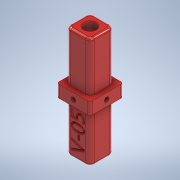
# Autodesk Inventor part: Supports
Saved by Autodesk Inventor 2020 (Build 240168000, 168)
## iProperties
Created: 2019-07-12
Part Number: Supports
Material: PBT Plastic
Document SubType Name: Modeling
Designer: steele
Density: 1.31 g/cm^3
Appearance: Orange-Red
Author: steele
Autodesk Inventor part; units mm, degrees
ref_plane "YZ Plane" through (0, 0, 0) normal (1, 0, 0) x (0, 1, 0)
ref_plane "XZ Plane" through (0, 0, 0) normal (0, 1, 0) x (-1, 0, 0)
ref_plane "XY Plane" through (0, 0, 0) normal (0, 0, 1) x (1, 0, 0)
sketch "Sketch1" plane through (0, 0, 0) normal (0, 1, 0) x (-1, 0, 0)
  line L0 (11.43, 11.43) -> (-11.43, 11.43)
  line L1 (-11.43, 11.43) -> (-11.43, -11.43)
  line L2 (-11.43, -11.43) -> (11.43, -11.43)
  line L3 (11.43, -11.43) -> (11.43, 11.43)
  line L4 (11.43, 11.43) -> (-11.43, -11.43) construction
  line L5 (-11.43, 11.43) -> (11.43, -11.43) construction
  point P0 (0, 0)
  dimension "outerWidth" = 22.86
  dimension "outerLength" = 22.86
  constraints: 12 end point, 2 midpoint, 2 parallel, 1 horizontal, 1 perpendicular
  measures "outerWidth" distance of L0.start L0.end
  measures "outerLength" distance of L1.end L0.end
extrude "CenterPortion" add sketch "Sketch1" along normal mid plane 8.382
sketch "Sketch2" plane through (0, 0, 0) normal (0, 1, 0) x (-1, 0, 0)
  line L0 (8.255, 8.255) -> (-8.255, 8.255)
  line L1 (-8.255, 8.255) -> (-8.255, -8.255)
  line L2 (-8.255, -8.255) -> (8.255, -8.255)
  line L3 (8.255, -8.255) -> (8.255, 8.255)
  line L4 (8.255, 8.255) -> (-8.255, -8.255) construction
  line L5 (-8.255, 8.255) -> (8.255, -8.255) construction
  point P0 (0, 0)
  dimension "innerWidth" = 16.51
  dimension "innerLength" = 16.51
  constraints: 12 end point, 2 midpoint, 2 parallel, 1 horizontal, 1 perpendicular
  measures "innerWidth" distance of L0.start L0.end
  measures "innerLength" distance of L1.end L0.end
extrude "OuterPortion" add sketch "Sketch2" along normal mid plane 76.2
sketch "Sketch3" plane through (-8.255, -4.191, 8.255) normal (0, 0, 1) x (1, 0, 0)
  line L0 (0, -33.909) -> (16.51, -33.909) construction
  line L1 (12.7, -33.909) -> (12.7, 0) construction
  line L2 (19.685, 0) -> (-3.175, 0) construction
  line L3 (16.51, -33.909) -> (16.51, 0) projected
  line L4 (3.81, -22.1451) -> (12.7, -25.2069)
  line L5 (12.7, -25.2069) -> (12.7, -26.4821)
  line L6 (12.7, -26.4821) -> (3.81, -29.5439)
  line L7 (3.81, -29.5439) -> (3.81, -28.2759)
  line L8 (3.81, -28.2759) -> (11.1943, -25.8121)
  line L9 (11.1943, -25.8121) -> (3.81, -23.3482)
  line L10 (3.81, -23.3482) -> (3.81, -22.1451)
  line L11 (9.35, -18.19) -> (9.35, -21.5544)
  line L12 (9.35, -21.5544) -> (8.2694, -21.5544)
  line L13 (8.2694, -21.5544) -> (8.2694, -18.19)
  line L14 (8.2694, -18.19) -> (9.35, -18.19)
  spline S0 degree 2 poles (8.255, -11.4757) (10.6468, -11.4757) (12.8873, -12.8661) (12.8873, -14.3142) knots 0 0 0 1 2 2 2
  spline S1 degree 2 poles (12.8873, -14.3142) (12.8873, -15.7838) (10.6036, -17.1598) (8.2622, -17.1598) knots 0 0 0 1 2 2 2
  spline S2 degree 2 poles (8.2622, -17.1598) (5.856, -17.1598) (3.6299, -15.7694) (3.6299, -14.3142) knots 0 0 0 1 2 2 2
  spline S3 degree 2 poles (3.6299, -14.3142) (3.6299, -12.8517) (5.9352, -11.4757) (8.255, -11.4757) knots 0 0 0 1 2 2 2
  spline S4 degree 2 poles (10.9638, -13.003) (10.5243, -12.8301) (9.1699, -12.686) (8.255, -12.686) knots 0 0 0 1 2 2 2
  spline S5 degree 2 poles (8.255, -12.686) (7.3401, -12.686) (5.9929, -12.8301) (5.539, -13.0102) knots 0 0 0 1 2 2 2
  spline S6 degree 2 poles (5.539, -13.0102) (5.0851, -13.1903) (4.6169, -13.8171) (4.6169, -14.3142) knots 0 0 0 1 2 2 2
  spline S7 degree 2 poles (4.6169, -14.3142) (4.6169, -14.8112) (5.0851, -15.4524) (5.5534, -15.6397) knots 0 0 0 1 2 2 2
  spline S8 degree 2 poles (5.5534, -15.6397) (6.0073, -15.8198) (7.3905, -15.9495) (8.2622, -15.9495) knots 0 0 0 1 2 2 2
  spline S9 degree 2 poles (8.2622, -15.9495) (9.1988, -15.9495) (10.4523, -15.8342) (10.9422, -15.6469) knots 0 0 0 1 2 2 2
  spline S10 degree 2 poles (10.9422, -15.6469) (11.4032, -15.474) (11.9003, -14.8329) (11.9003, -14.3142) knots 0 0 0 1 2 2 2
  spline S11 degree 2 poles (11.9003, -14.3142) (11.9003, -13.8243) (11.4321, -13.1831) (10.9638, -13.003) knots 0 0 0 1 2 2 2
  spline S12 degree 2 poles (9.8759, -4.9487) (10.5171, -4.9487) (11.6122, -5.3593) (12.0156, -5.7339) knots 0 0 0 1 2 2 2
  spline S13 degree 2 poles (12.0156, -5.7339) (12.419, -6.1086) (12.8873, -7.2252) (12.8873, -7.9168) knots 0 0 0 1 2 2 2
  spline S14 degree 2 poles (12.8873, -7.9168) (12.8873, -8.5508) (12.6063, -9.7899) (12.383, -10.2438) knots 0 0 0 1 2 2 2
  line L15 (12.383, -10.2438) -> (11.1223, -10.2438)
  line L16 (11.1223, -10.2438) -> (11.1223, -10.1573)
  spline S15 degree 2 poles (11.1223, -10.1573) (11.2231, -10.0204) (11.4825, -9.5089) (11.5978, -9.1992) knots 0 0 0 1 2 2 2
  spline S16 degree 2 poles (11.5978, -9.1992) (11.7202, -8.8462) (11.8571, -8.2626) (11.8571, -7.8952) knots 0 0 0 1 2 2 2
  spline S17 degree 2 poles (11.8571, -7.8952) (11.8571, -7.535) (11.5978, -6.8578) (11.3168, -6.6129) knots 0 0 0 1 2 2 2
  spline S18 degree 2 poles (11.3168, -6.6129) (11.0502, -6.3895) (10.3442, -6.159) (9.8687, -6.159) knots 0 0 0 1 2 2 2
  spline S19 degree 2 poles (9.8687, -6.159) (9.3933, -6.159) (8.7881, -6.4183) (8.5864, -6.6633) knots 0 0 0 1 2 2 2
  spline S20 degree 2 poles (8.5864, -6.6633) (8.3631, -6.9154) (8.1758, -7.6647) (8.1758, -8.1185) knots 0 0 0 1 2 2 2
  spline S21 degree 2 poles (8.1758, -8.1185) (8.1758, -8.6084) (8.327, -9.581) (8.3919, -9.8764) knots 0 0 0 1 2 2 2
  line L17 (8.3919, -9.8764) -> (3.81, -9.8764)
  line L18 (3.81, -9.8764) -> (3.81, -4.9991)
  line L19 (3.81, -4.9991) -> (4.8546, -4.9991)
  line L20 (4.8546, -4.9991) -> (4.8546, -8.7309)
  line L21 (4.8546, -8.7309) -> (7.2248, -8.7309)
  spline S22 degree 2 poles (7.2248, -8.7309) (7.196, -8.5148) (7.1744, -8.0969) (7.1744, -7.924) knots 0 0 0 1 2 2 2
  spline S23 degree 2 poles (7.1744, -7.924) (7.1744, -7.2396) (7.3977, -6.2959) (7.7291, -5.8636) knots 0 0 0 1 2 2 2
  spline S24 degree 2 poles (7.7291, -5.8636) (8.0605, -5.4242) (9.0691, -4.9487) (9.8759, -4.9487) knots 0 0 0 1 2 2 2
  point P0 (8.255, 4.191)
  dimension "textCenterLine" = 3.81
  constraints: 2 end point, 2 point on line, 2 vertical
  measures "textCenterLine" distance between parallel lines of L3 L1
extrude "TextWithVersionNumber" cut sketch "Sketch3" against normal blind 2.54
sketch "Sketch4" plane through (0, 38.1, 0) normal (0, 1, 0) x (1, 0, 0)
  point P0 (0, 0)
  point P1 (0, 0)
  constraints: 1 coincident
hole "CenterSupportHole" at (0, 38.1, 0) direction (0, -1, 0) diameter 8.89 end through all
fillet "Fillet1" radius 1.5875 4 edges at (-11.43, 0, 11.43) (11.43, 0, 11.43) (11.43, 0, -11.43) (-11.43, 0, -11.43)
fillet "Fillet2" radius 3.175 8 edges at (8.255, 21.1455, -8.255) (8.255, 21.1455, 8.255) (-8.255, 21.1455, -8.255) (-8.255, 21.1455, 8.255) (8.255, -21.1455, -8.255) (8.255, -21.1455, 8.255) (-8.255, -21.1455, -8.255) (-8.255, -21.1455, 8.255)
sketch "Sketch5" plane through (-9.8425, 4.191, 11.43) normal (0, 0, 1) x (1, 0, 0)
  point P0 (9.8425, -4.191)
  point P1 (9.8425, -4.191)
  constraints: 1 coincident
sketch "Sketch6" plane through (11.43, -4.191, -9.8425) normal (1, 0, 0) x (0, 0, -1)
  point P0 (-9.8425, 4.191)
  point P1 (-9.8425, 4.191)
  constraints: 1 coincident
sketch "Sketch7" plane through (9.8425, 4.191, -11.43) normal (0, 0, -1) x (-1, 0, 0)
  point P0 (9.8425, -4.191)
  point P1 (9.8425, -4.191)
  constraints: 1 coincident
sketch "Sketch8" plane through (-11.43, -4.191, -9.8425) normal (-1, 0, 0) x (0, 0, 1)
  point P0 (9.8425, 4.191)
  point P1 (9.8425, 4.191)
  constraints: 1 coincident
hole "Hole2" at (0, 0, 11.43) direction (0, 0, -1) diameter 3.048 depth 12.7 tip angle 118
hole "Hole3" at (11.43, 0, 0) direction (-1, 0, 0) diameter 3.048 depth 12.7 tip angle 118
hole "Hole4" at (0, 0, -11.43) direction (0, 0, 1) diameter 3.048 depth 12.7 tip angle 118
hole "Hole5" at (-11.43, 0, 0) direction (1, 0, 0) diameter 3.048 depth 12.7 tip angle 118
fillet "BottomFillet" radius 1.5875 8 edges at (0, -38.1, 8.255) (7.3251, -38.1, 7.3251) (8.255, -38.1, 0) (7.3251, -38.1, -7.3251) (0, -38.1, -8.255) (-7.3251, -38.1, -7.3251) (-8.255, -38.1, 0) (-7.3251, -38.1, 7.3251)
fillet "TopFille" radius 1.5875 8 edges at (-7.3251, 38.1, 7.3251) (0, 38.1, 8.255) (7.3251, 38.1, 7.3251) (8.255, 38.1, 0) (7.3251, 38.1, -7.3251) (0, 38.1, -8.255) (-7.3251, 38.1, -7.3251) (-8.255, 38.1, 0)
equation "\"textCenterLine\" = 0.5 * innerWidth - 0.5 * textHeight"
equation "\"textHeight\" = 8.89"
body "Solid1"
